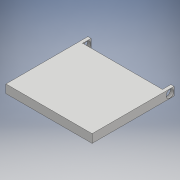
# Autodesk Inventor part: mesa
Saved by Autodesk Inventor 2018 (Build 220112000, 112)
## iProperties
Created: 2018-01-13
Part Number: mesa
Material: Generic
Document SubType Name: Modeling
Designer: mokuz
Density: 1 g/cm^3
Appearance: Default
Author: mokuz
Autodesk Inventor part; units mm, degrees
ref_plane "YZ Plane" through (0, 0, 0) normal (1, 0, 0) x (0, 1, 0)
ref_plane "XZ Plane" through (0, 0, 0) normal (0, 1, 0) x (-1, 0, 0)
ref_plane "XY Plane" through (0, 0, 0) normal (0, 0, 1) x (1, 0, 0)
sketch "Sketch1" plane through (0, 0, 0) normal (0, 0, 1) x (1, 0, 0)
  line L0 (0, 0) -> (820, 0)
  line L1 (820, 0) -> (820, 700)
  line L2 (820, 700) -> (0, 700)
  line L3 (0, 700) -> (0, 0)
  dimension "d0" = 820
  dimension "d1" = 700
  constraints: 8 end point, 2 parallel, 1 horizontal, 1 perpendicular
  measures "d0" distance of L2.end L1.end
  measures "d1" distance of L1.end L0.end
extrude "Extrusion1" add sketch "Sketch1" along normal blind 80
sketch "Sketch2" plane through (820, 0, 0) normal (1, 0, 0) x (0, 0, -1)
  line L0 (0, 0) -> (0, 700) projected
  line L1 (0, 700) -> (-80, 700) projected
  line L2 (-80, 0) -> (-80, 700) projected
  line L3 (0, 0) -> (-80, 0) projected
  line L4 (0, 0) -> (0, 700) projected
  line L5 (0, 700) -> (-80, 700)
  line L6 (-80, 700) -> (-80, 780)
  line L7 (-80, 780) -> (0, 780)
  line L8 (0, 780) -> (0, 700)
  dimension "d4" = 80
  dimension "d5" = 80
  constraints: 8 end point, 2 parallel, 1 horizontal, 1 perpendicular
  measures "d4" distance of L6.end L7.end
  measures "d5" distance of L5.end L6.end
extrude "Extrusion2" add sketch "Sketch2" against normal blind 30 contours L1 L6 L7 L8
sketch "Sketch3" plane through (0, 0, 0) normal (-1, 0, 0) x (0, 0, 1)
  line L0 (0, 700) -> (0, 0) projected
  line L1 (0, 0) -> (80, 0) projected
  line L2 (80, 700) -> (80, 0) projected
  line L3 (0, 700) -> (80, 700) projected
  line L4 (0, 780) -> (0, 700) projected
  line L5 (80, 700) -> (0, 700) projected
  line L6 (80, 700) -> (80, 780) projected
  line L7 (80, 780) -> (0, 780) projected
  line L8 (80, 0) -> (80, 780) projected
  line L9 (0, 700) -> (80, 700)
  line L10 (80, 700) -> (80, 780)
  line L11 (80, 780) -> (0, 780)
  line L12 (0, 780) -> (0, 700)
  point P0 (72, 700)
  constraints: 8 end point, 2 parallel, 1 horizontal, 1 perpendicular, 1 other
extrude "Extrusion3" add sketch "Sketch3" against normal blind 30 contours L4 L7 L6 L3
sketch "Sketch4" plane through (0, 0, 0) normal (-1, 0, 0) x (0, 0, 1)
  line L0 (0, 780) -> (80, 780) projected
  line L1 (80, 780) -> (80, 700) projected
  line L2 (0, 700) -> (80, 700) projected
  line L3 (0, 700) -> (0, 780) projected
  circle A0 centre (40, 740) radius 36.5
  point P0 (0, 0)
  dimension "d10" = 73
  constraints: 1 centre point
  measures "d10" diameter of A0
extrude "Extrusion4" cut sketch "Sketch4" against normal blind 940.75 contours A0
body "Solid1"
